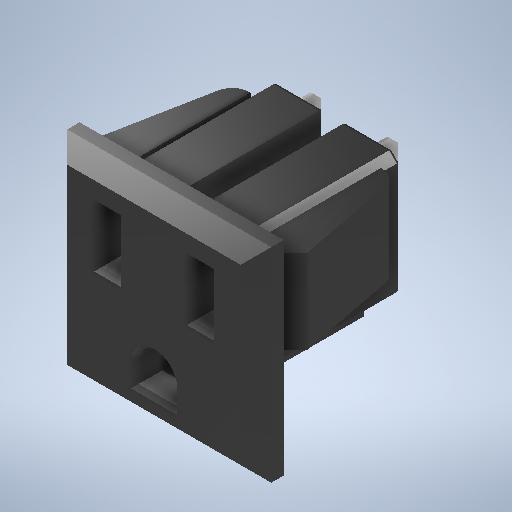
# Autodesk Inventor part: Plug
Saved by Autodesk Inventor 2025 (Build 290162000, 162)
## iProperties
Created: 2024-08-08
Part Number: Plug
Material: Generic
Document SubType Name: Modeling
Designer: ethan
Density: 1 g/cm^3
Appearance: Default
Author: ethan
Autodesk Inventor part; units mm, degrees
ref_plane "YZ Plane" through (0, 0, 0) normal (1, 0, 0) x (0, 1, 0)
ref_plane "XZ Plane" through (0, 0, 0) normal (0, 1, 0) x (-1, 0, 0)
ref_plane "XY Plane" through (0, 0, 0) normal (0, 0, 1) x (1, 0, 0)
sketch "Sketch1" plane through (0, 0, 0) normal (0, 0, 1) x (1, 0, 0)
  line L0 (0, 0) -> (26.6, 0)
  line L1 (26.6, 0) -> (26.6, 26.6)
  line L2 (26.6, 26.6) -> (0, 26.6)
  line L3 (0, 26.6) -> (0, 0)
  dimension "d0" = 26.6
  dimension "d1" = 26.6
  constraints: 8 end point, 2 parallel, 1 horizontal, 1 perpendicular
  measures "d0" distance of L2.end L1.end
  measures "d1" distance of L1.end L0.end
extrude "Extrusion1" add sketch "Sketch1" along normal blind 3.6
chamfer "Chamfer1" distance 2 angle 45 4 edges at (13.3, 26.6, 0) (0, 13.3, 0) (26.6, 13.3, 0) (13.3, 0, 0)
sketch "Sketch2" plane through (0, 0, 0) normal (0, 0, -1) x (-1, 0, 0)
  line L0 (0, 26.6) -> (0, 0) construction
  line L1 (0, 20.5614) -> (-6, 20.5614) construction
  line L2 (-26.6, 26.6) -> (0, 26.6) construction
  line L3 (-7.1317, 26.6) -> (-7.1317, 21.9) construction
  line L4 (-7.1317, 26.6) -> (-2.4317, 26.6) construction
  line L5 (-6, 21.9) -> (-8.5, 21.9) construction
  line L6 (-8.5, 21.9) -> (-8.5, 14.8) construction
  line L7 (-8.5, 14.8) -> (-6, 14.8) construction
  line L8 (-6, 14.8) -> (-6, 21.9) construction
  line L9 (-13.3, 26.6) -> (-13.3, 0) construction
  line L10 (0, 0) -> (-26.6, 0) construction
  line L11 (-20.6, 21.9) -> (-18.1, 21.9) construction
  line L12 (-18.1, 21.9) -> (-18.1, 14.8) construction
  line L13 (-18.1, 14.8) -> (-20.6, 14.8) construction
  line L14 (-20.6, 14.8) -> (-20.6, 21.9) construction
  line L15 (-13.3, 0) -> (-13.3, 4) construction
  line L16 (-13.3, 4) -> (-10.8, 4) construction
  line L17 (-10.8, 4) -> (-15.8, 4) construction
  line L18 (-15.8, 4) -> (-15.8, 9) construction
  line L19 (-15.8, 9) -> (-10.8, 9) construction
  line L20 (-10.8, 9) -> (-10.8, 4) construction
  line L21 (-15.8, 4) -> (-15.8, 7) construction
  line L22 (-10.8, 4) -> (-10.8, 7) construction
  arc A0 (-10.8, 7) -> (-15.8, 7) centre (-13.3, 6.4375) ccw construction
  line L23 (-20.6, 21.9) -> (-18.1, 21.9)
  line L24 (-18.1, 21.9) -> (-18.1, 14.8)
  line L25 (-18.1, 14.8) -> (-20.6, 14.8)
  line L26 (-20.6, 14.8) -> (-20.6, 21.9)
  line L27 (-8.5, 21.9) -> (-6, 21.9)
  line L28 (-6, 21.9) -> (-6, 14.8)
  line L29 (-6, 14.8) -> (-8.5, 14.8)
  line L30 (-8.5, 14.8) -> (-8.5, 21.9)
  line L31 (-15.8, 4) -> (-10.8, 4)
  line L32 (-10.8, 7) -> (-10.8, 4)
  line L33 (-15.8, 4) -> (-15.8, 7)
  arc A1 (-10.8, 7) -> (-15.8, 7) centre (-13.3, 6.4375) ccw
  dimension "d7" = 6
  dimension "d9" = 4.7
  dimension "d11" = 2.5
  dimension "d12" = 7.1
  dimension "d13" = 4
  dimension "d14" = 2.5
  dimension "d15" = 5
  dimension "d16" = 5
  dimension "d17" = 3
  constraints: 62 end point, 8 parallel, 8 perpendicular, 5 horizontal, 5 point on line, 4 point on circle, 4 symmetric about line, 3 collinear, 2 centre point, 2 midpoint, 1 concentric
  measures "d7" distance of L1.start L1.end
  measures "d9" distance of L3.start L3.end
  measures "d11" distance of L7.end L6.end
  measures "d12" distance of L6.end L5.end
  measures "d13" distance of L9.end L15.end
  measures "d14" distance of L15.end L16.end
  measures "d15" distance of L18.end L19.end
  measures "d16" distance of L17.end L18.end
  measures "d17" distance of L17.end L21.end
extrude "Extrusion2" cut sketch "Sketch2" against normal blind 3.6
sketch "Sketch3" plane through (0, 0, 3.6) normal (0, 0, 1) x (1, 0, 0)
  line L0 (15.8, 4) -> (10.8, 4) construction
  line L1 (10.8, 4) -> (10.8, 7) construction
  arc A0 (15.8, 7) -> (10.8, 7) centre (13.3, 6.4375) ccw construction
  line L2 (15.8, 7) -> (15.8, 4) construction
  line L3 (6, 14.8) -> (6, 21.9) construction
  line L4 (6, 21.9) -> (8.5, 21.9) construction
  line L5 (8.5, 21.9) -> (8.5, 14.8) construction
  line L6 (8.5, 14.8) -> (6, 14.8) construction
  line L7 (18.1, 14.8) -> (18.1, 21.9) construction
  line L8 (18.1, 21.9) -> (20.6, 21.9) construction
  line L9 (20.6, 21.9) -> (20.6, 14.8) construction
  line L10 (20.6, 14.8) -> (18.1, 14.8) construction
  line L11 (26.6, 0) -> (26.6, 26.6) construction
  line L12 (26.6, 26.6) -> (0, 26.6) construction
  line L13 (0, 26.6) -> (0, 0) construction
  line L14 (0, 0) -> (26.6, 0) construction
  line L15 (13.3, 26.6) -> (13.3, 0) construction
  line L16 (4.8, 2.55) -> (21.8, 2.55) construction
  line L17 (21.8, 2.55) -> (21.8, 24.05) construction
  line L18 (21.8, 24.05) -> (4.8, 24.05) construction
  line L19 (4.8, 24.05) -> (4.8, 2.55) construction
  line L20 (4.8, 2.55) -> (21.8, 24.05) construction
  line L21 (21.8, 2.55) -> (4.8, 24.05) construction
  line L22 (21.8, 2.55) -> (17.4, 2.55) construction
  line L23 (17.4, 2.55) -> (17.4, 8.55) construction
  line L24 (17.4, 8.55) -> (21.8, 8.55) construction
  line L25 (21.8, 8.55) -> (21.8, 2.55) construction
  line L26 (4.8, 2.55) -> (9.2, 2.55) construction
  line L27 (9.2, 2.55) -> (9.2, 8.55) construction
  line L28 (9.2, 8.55) -> (4.8, 8.55) construction
  line L29 (4.8, 8.55) -> (4.8, 2.55) construction
  line L30 (11.8, 37.0426) -> (14.8, 37.0426) construction
  line L31 (14.8, 37.0426) -> (14.8, 11.0574) construction
  line L32 (14.8, 11.0574) -> (11.8, 11.0574) construction
  line L33 (11.8, 11.0574) -> (11.8, 37.0426) construction
  line L34 (11.8, 37.0426) -> (14.8, 11.0574) construction
  line L35 (14.8, 37.0426) -> (11.8, 11.0574) construction
  line L36 (4.8, 24.05) -> (11.8, 24.05)
  line L37 (11.8, 11.0574) -> (11.8, 24.05)
  line L38 (11.8, 11.0574) -> (14.8, 11.0574)
  line L39 (14.8, 11.0574) -> (14.8, 24.05)
  line L40 (14.8, 24.05) -> (21.8, 24.05)
  line L41 (21.8, 24.05) -> (21.8, 8.55)
  line L42 (21.8, 8.55) -> (17.4, 8.55)
  line L43 (17.4, 8.55) -> (17.4, 2.55)
  line L44 (17.4, 2.55) -> (9.2, 2.55)
  line L45 (9.2, 2.55) -> (9.2, 8.55)
  line L46 (9.2, 8.55) -> (4.8, 8.55)
  line L47 (4.8, 8.55) -> (4.8, 24.05)
  point P0 (13.3, 13.3)
  point P1 (13.3, 24.05)
  dimension "d20" = 17
  dimension "d21" = 21.5
  dimension "d22" = 4.4
  dimension "d23" = 6
  dimension "d24" = 4.4
  dimension "d25" = 6
  dimension "d26" = 3
  constraints: 66 end point, 10 midpoint, 8 parallel, 8 perpendicular, 6 collinear, 3 horizontal
  measures "d20" distance of L18.end L17.end
  measures "d21" distance of L17.end L16.end
  measures "d22" distance of L23.end L24.end
  measures "d23" distance of L22.end L23.end
  measures "d24" distance of L28.end L27.end
  measures "d25" distance of L27.end L26.end
  measures "d26" distance of L30.start L30.end
extrude "Extrusion3" add sketch "Sketch3" along normal blind 20
chamfer "Chamfer2" distance 1 angle 45 4 edges at (4.8, 24.05, 13.6) (21.8, 24.05, 13.6) (17.4, 2.55, 13.6) (9.2, 2.55, 13.6)
fillet "Fillet1" radius 0.5 13 edges at (8.8, 24.05, 23.6) (4.8, 15.8, 23.6) (11.8, 17.5537, 23.6) (14.8, 17.5537, 23.6) (17.8, 24.05, 23.6) (21.8, 15.8, 23.6) (19.6, 8.55, 23.6) (17.4, 6.05, 23.6) (9.2, 6.05, 23.6) (7, 8.55, 23.6) (13.3, 2.55, 23.6) (21.3, 23.55, 23.6) (5.3, 23.55, 23.6)
sketch "Sketch4" plane through (14.8, 16.3, 3.6) normal (0, 1, 0) x (1, 0, 0)
  line L0 (-10, 0) -> (-10, -19.5) construction
  line L1 (11.8, 0) -> (-14.8, 0) construction
  line L2 (-8.7929, -20) -> (-3.5, -20) construction
  arc A0 (-3.5, -20) -> (-3, -19.5) centre (-3.5, -19.5) ccw construction
  line L3 (-3, -19.5) -> (-9, -19.5) construction
  ellipse E0 centre (-8.7929, -19.5) end of major axis (-8.7929, -20) minor radius 0.2071 (-9, -19.5) -> (-8.7929, -20) ccw construction
  line L4 (-9.5, -20) -> (-8.7929, -20) construction
  ellipse E1 centre (-8.7929, -19.5) end of major axis (-8.7929, -20) minor radius 0.2071 (-9, -19.5) -> (-8.7929, -20) ccw construction
  line L5 (-9, -19.5) -> (-10, -19.5) construction
  arc A1 (-10, -19.5) -> (-9.5, -20) centre (-9.5, -19.5) ccw construction
  line L6 (-7.8516, -20) -> (-7.8516, -17.5) construction
  line L7 (-7.8516, -17.5) -> (-16.9269, -17.5) construction
  line L8 (-10, -3.8087) -> (-15, -3.8087) construction
  line L9 (-14.8, 0) -> (-14.8, -3) construction
  line L10 (-10, 0) -> (-11.6, 0) construction
  line L11 (-11.6, 0) -> (-14.8, -3) construction
  line L12 (-10, -17.5) -> (-12, -17.5) construction
  line L13 (-12, -17.5) -> (-14.8, -3) construction
  arc A2 (-12.3892, -15.4843) -> (-10, -17.5) centre (-10.1078, -15.204) ccw construction
  arc A3 (-12.3892, -15.4843) -> (-10, -17.5) centre (-10.1078, -15.204) ccw
  line L14 (-12.3892, -15.4843) -> (-14.8, -3)
  line L15 (-14.8, -3) -> (-11.6, 0)
  line L16 (-11.6, 0) -> (-10, 0)
  line L17 (-10, 0) -> (-10, -17.5)
  point P0 (-14.8, 3.6)
  dimension "d33" = 2.5
  dimension "d34" = 5
  dimension "d35" = 3
  dimension "d36" = 1.6
  dimension "d37" = 2
  constraints: 24 end point, 7 point on line, 4 point on circle, 3 collinear, 2 centre point, 2 vertical, 1 concentric, 1 horizontal, 1 perpendicular, 2 other
  measures "d33" distance of L6.start L6.end
  measures "d34" distance of L8.start L8.end
  measures "d35" distance of L1.end L9.end
  measures "d36" distance of L0.start L10.end
  measures "d37" distance of L12.start L12.end
extrude "Extrusion4" add sketch "Sketch4" along normal blind 7.3 and the other way blind 3.65
mirror "Mirror1" about plane through (13.3, 11.0574, 3.6) normal (-1, 0, 0) of "Extrusion4"
ref_plane "LeftLine" through (8.3, 11.0574, 3.6) normal (1, 0, 0) x (0, 0, -1)
sketch "Sketch5" plane through (8.3, 11.0574, 3.6) normal (1, 0, 0) x (0, 0, -1)
  line L0 (-20, -2.0074) -> (-20, 11.7855) construction
  line L1 (-19.5, 12.9926) -> (0, 12.9926) construction
  line L2 (-20, 11.7855) -> (-20, 12.4926) construction
  line L3 (0, -2.5074) -> (-19.5, -2.5074) construction
  line L4 (-20, 12.9926) -> (-13.6632, 12.9926) construction
  line L5 (-13.6632, 12.9926) -> (-13.6632, -2.5074) construction
  line L6 (-13.6632, -2.5074) -> (-20, -2.5074) construction
  line L7 (-20, -2.5074) -> (-20, 12.9926) construction
  line L8 (-20, 12.9926) -> (-20, 11.9926) construction
  line L9 (-20, -2.5074) -> (-20, 2.4926) construction
  line L10 (-20, 2.4926) -> (-23, 2.4926) construction
  line L11 (-23, 2.4926) -> (-23, 11.9926) construction
  line L12 (-23, 11.9926) -> (-20, 11.9926) construction
  line L13 (-20, 11.9926) -> (-20, 2.4926) construction
  line L14 (-23, 11.9926) -> (-20, 11.9926)
  line L15 (-20, 11.9926) -> (-20, 2.4926)
  line L16 (-20, 2.4926) -> (-23, 2.4926)
  line L17 (-23, 2.4926) -> (-23, 11.9926)
  point P0 (3.6, -11.0574)
  dimension "d42" = 1
  dimension "d43" = 5
  dimension "d44" = 3
  constraints: 28 end point, 6 parallel, 3 horizontal, 3 perpendicular, 3 point on line
  measures "d42" distance of L4.start L8.end
  measures "d43" distance of L6.end L9.end
  measures "d44" distance of L11.end L12.end
extrude "Extrusion5" add sketch "Sketch5" along normal mid plane 0.35
chamfer "Chamfer3" distance 1 angle 45 2 edges at (8.3, 23.05, 26.6) (8.3, 13.55, 26.6)
mirror "Mirror2" about plane through (13.3, 11.0574, 3.6) normal (-1, 0, 0) of "Extrusion5", "Chamfer3"
chamfer "Chamfer4" distance 0.5 angle 45 12 edges at (19.35, 21.9, 0) (18.1, 18.35, 0) (20.6, 18.35, 0) (19.35, 14.8, 0) (7.25, 14.8, 0) (6, 18.35, 0) (7.25, 21.9, 0) (8.5, 18.35, 0) (13.3, 9, 0) (15.8, 5.5, 0) (10.8, 5.5, 0) (13.3, 4, 0)
body "Solid1"
